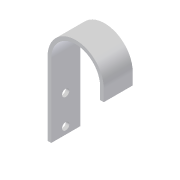
# Autodesk Inventor part: FE-00016
Saved by Autodesk Inventor 2012 (Build 160160000, 160)
## iProperties
Company: FIRST
Created: 2008-05-30
Part Number: FE-00016
Document SubType Name: Modeling
Designer: dfoster
Density: 1 g/cm^3
Description: Hanger, Plastic
Mass: 11.6479 g
Surface Area: 85.5823 cm^2
Volume: 11.6479 cm^3
Material: Default
Title: Hanger, Plastic
Author: dfoster
Autodesk Inventor part; units mm, degrees
ref_plane "YZ Plane" through (0, 0, 0) normal (1, 0, 0) x (0, 1, 0)
ref_plane "XZ Plane" through (0, 0, 0) normal (0, 1, 0) x (-1, 0, 0)
ref_plane "XY Plane" through (0, 0, 0) normal (0, 0, 1) x (1, 0, 0)
sketch "Sketch1" plane through (0, 0, 0) normal (0, 0, 1) x (1, 0, 0)
  line L0 (-42.8625, -38.1) -> (-42.8625, 26.1937)
  arc A0 (6.35, 26.1938) -> (-42.8625, 26.1937) centre (-18.2562, 26.1937) ccw
  line L1 (6.35, 26.1938) -> (6.35, 15.875)
  line L2 (-39.6875, -38.1) -> (-39.6875, 26.1937)
  arc A1 (3.175, 26.1938) -> (-39.6875, 26.1937) centre (-18.2562, 26.1937) ccw
  line L3 (3.175, 26.1938) -> (3.175, 15.875)
  line L4 (-42.8625, -38.1) -> (-39.6875, -38.1)
  line L5 (3.175, 15.875) -> (6.35, 15.875)
  dimension "d0" = 3.175
  dimension "d1" = 88.9
  dimension "d2" = 21.4312
  dimension "d3" = 34.925
  constraints: 12 end point, 4 point on circle, 3 parallel, 2 centre point, 2 tangent, 1 perpendicular, 1 vertical, 2 other
  measures "d0" distance of L3.end L1.end
  measures "d2" radius of A1
extrude "Extrusion1" add sketch "Sketch1" along normal blind 25.4
hole "Hole1" at (-39.6875, -31.75, 12.7) direction (-1, 0, 0) diameter 6.35 end through all
pattern_linear "Rectangular Pattern1" count 2 spacing 25.4 along (0, 1, 0) of "Hole1"
body "Solid1"
